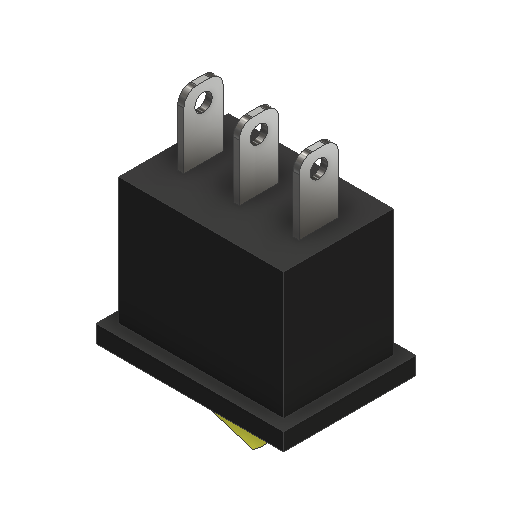
# Autodesk Inventor part: COTS_GENERIC_AC_Power_Switch_5A
Saved by Autodesk Inventor 2026.1 (Build 301233000, 233)
## iProperties
Created: 2016-06-26
Part Number: COTS_GENERIC_AC_Power_Switch_5A
Material: Ogólny
Document SubType Name: Modeling
Designer: Andrzej
Density: 1 g/cm^3
Appearance: Kauczuk - czarny
Mass: 4.45746 g
Surface Area: 20.2954 cm^2
Volume: 4.45746 cm^3
Author: Andrzej
Autodesk Inventor part; units mm, degrees
ref_plane "YZ Plane" through (0, 0, 0) normal (1, 0, 0) x (0, 1, 0)
ref_plane "XZ Plane" through (0, 0, 0) normal (0, 1, 0) x (-1, 0, 0)
sketch "Szkic1" plane through (0, 0, 0) normal (0, 0, 1) x (1, 0, 0)
  line L0 (-6.6876, 6.2431) -> (12.1124, 6.2431)
  line L1 (12.1124, 6.2431) -> (12.1124, -6.2569)
  line L2 (12.1124, -6.2569) -> (-6.6876, -6.2569)
  line L3 (-6.6876, -6.2569) -> (-6.6876, 6.2431)
  line L4 (-3.9802, 2.2431) -> (-3.2802, 2.2431)
  line L5 (-3.2802, 2.2431) -> (-3.2802, -2.2569)
  line L6 (-3.2802, -2.2569) -> (-3.9802, -2.2569)
  line L7 (-3.9802, -2.2569) -> (-3.9802, 2.2431)
  line L8 (2.3508, 2.2431) -> (3.0508, 2.2431)
  line L9 (3.0508, 2.2431) -> (3.0508, -2.2569)
  line L10 (3.0508, -2.2569) -> (2.3508, -2.2569)
  line L11 (2.3508, -2.2569) -> (2.3508, 2.2431)
  line L12 (9.1799, 2.2431) -> (9.8799, 2.2431)
  line L13 (9.8799, 2.2431) -> (9.8799, -2.2569)
  line L14 (9.8799, -2.2569) -> (9.1799, -2.2569)
  line L15 (9.1799, -2.2569) -> (9.1799, 2.2431)
  point P0 (0, 0)
  dimension "d0" = 18.8
  dimension "d1" = 12.5
  dimension "d2" = 0.7
  dimension "d3" = 4.5
  dimension "d4" = 4
  dimension "d5" = 0.7
  dimension "d6" = 4.5
  dimension "d7" = 0.7
  dimension "d8" = 4.5
  constraints: 32 end point, 8 parallel, 4 horizontal, 4 perpendicular
  measures "d0" distance of L1.end L2.end
  measures "d1" distance of L0.end L1.end
  measures "d2" distance of L5.end L6.end
  measures "d3" distance of L6.end L4.start
  measures "d4" distance between parallel lines of L0 L4
  measures "d5" distance of L9.end L10.end
  measures "d6" distance of L10.end L8.start
  measures "d7" distance of L13.end L14.end
  measures "d8" distance of L14.end L12.start
extrude "Wyciągnięcie proste1" add sketch "Szkic1" against normal blind 14.5 contours L0 L1 L2 L3 | L4 L5 L6 L7 | L8 L9 L10 L11 | L12 L13 L14 L15
extrude "Wyciągnięcie proste2" add sketch "Szkic1" along normal blind 8 contours L4 L5 L6 L7 | L8 L9 L10 L11 | L12 L13 L14 L15
fillet "Zaokrąglenie1" radius 1.5 6 edges at (-3.6302, 2.2431, 8) (2.7008, 2.2431, 8) (9.5299, 2.2431, 8) (-3.6302, -2.2569, 8) (2.7008, -2.2569, 8) (9.5299, -2.2569, 8)
sketch "Szkic2" plane through (0, 0, -14.5) normal (0, 0, -1) x (-1, 0, 0)
  line L0 (6.6876, 6.2431) -> (-12.1124, 6.2431) projected
  line L1 (-12.1124, 6.2431) -> (-12.1124, -6.2569) projected
  line L2 (-12.1124, -6.2569) -> (6.6876, -6.2569) projected
  line L3 (6.6876, -6.2569) -> (6.6876, 6.2431) projected
  line L4 (-13.4124, 7.5431) -> (7.9876, 7.5431)
  line L5 (7.9876, 7.5431) -> (7.9876, -7.5569)
  line L6 (7.9876, -7.5569) -> (-13.4124, -7.5569)
  line L7 (-13.4124, -7.5569) -> (-13.4124, 7.5431)
  point P0 (0, 0)
  dimension "d14" = 18.8
  dimension "d15" = 1.3
  constraints: 8 end point, 3 other
  measures "d14" distance between parallel lines of L3 L1
  measures "d15" distance between parallel lines of L0 L4
extrude "Wyciągnięcie proste3" add sketch "Szkic2" along normal blind 2 contours L3 L2 L1 L0 | L4 L5 L6 L7
sketch "Szkic3" plane through (-3.9802, -2.2569, 0) normal (-1, 0, 0) x (0, 0, 1)
  line L0 (0, 4.5) -> (6.5, 4.5) projected
  line L1 (0, 0) -> (6.5, 0) projected
  point P0 (0, 2.2569)
  point P1 (5.956, 2.25)
  dimension "d18" = 4.5
  dimension "d19" = 2.25
  measures "d18" distance between parallel lines of L0 L1
  measures "d19" distance from line of L0 point (5.956, 2.25)
hole "Otwór1" at (-3.9802, -0.0069, 5.956) direction (1, 0, 0) diameter 2 end through all
ref_plane "Płaszczyzna konstrukcyjna1" through (-7.9876, -5.0569, -14.5) normal (0, -1, 0) x (1, 0, 0)
sketch "Szkic4" plane through (-7.9876, -5.0569, -14.5) normal (0, -1, 0) x (1, 0, 0)
  line L0 (21.4, 0) -> (0, 0) projected
  line L1 (21.4, 0) -> (21.4, -2) projected
  line L2 (0, -2) -> (21.4, -2) projected
  line L3 (0, 0) -> (0, -2) projected
  line L4 (0, -2) -> (21.4, -2) projected
  arc A0 (15.4, -6) -> (18.4, -2) centre (11.6248, -0.0436) ccw
  line L5 (15.4, -6) -> (2.5, -2)
  point P0 (7.9876, 14.5)
  dimension "d28" = 3
  dimension "d29" = 2.5
  dimension "d30" = 4
  dimension "d31" = 6
  constraints: 2 end point, 2 point on circle, 2 point on line, 1 centre point
  measures "d28" distance from line of L1 A0.end
  measures "d29" distance from line of L3 L5.end
  measures "d30" distance from line of L5.start L2
  measures "d31" distance from line of L5.start L1
extrude "Wyciągnięcie proste4" add sketch "Szkic4" against normal blind 10.1 contours A0 L5 L2
sketch "Szkic5" plane through (-5.4876, -5.0569, -16.5) normal (-0.2962, 0, -0.9551) x (-0.9551, 0, 0.2962)
  line L0 (-13.2267, 2.4266) -> (-13.2267, 8.6477) construction
  line L1 (-13.2267, 8.6477) -> (-8.9095, 8.6477) construction
  line L2 (-8.9095, 8.6477) -> (-8.9095, 2.4266) construction
  line L3 (-8.9095, 2.4266) -> (-13.2267, 2.4266) construction
  line L4 (-6.957, 3.6505) -> (-6.957, 6.2802) construction
  line L5 (-6.957, 6.2802) -> (-0.4173, 6.2802) construction
  line L6 (-0.4173, 6.2802) -> (-0.4173, 3.6505) construction
  line L7 (-0.4173, 3.6505) -> (-6.957, 3.6505) construction
  constraints: 4 other
equation "\"d4\" = -0.5 * d3 + 0.5 * d1"
equation "\"d19\" = 0.5 * d18"
